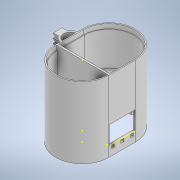
# Autodesk Inventor part: base-final
Saved by Autodesk Inventor 2021 (Build 250183000, 183)
## iProperties
Created: 2021-01-26
Part Number: base-final
Material: Generic
Document SubType Name: Modeling
Designer: Kayla
Density: 1 g/cm^3
Appearance: Default
Author: Kayla
Autodesk Inventor part; units mm, degrees
ref_plane "YZ Plane" through (0, 0, 0) normal (1, 0, 0) x (0, 1, 0)
ref_plane "XZ Plane" through (0, 0, 0) normal (0, 1, 0) x (-1, 0, 0)
ref_plane "XY Plane" through (0, 0, 0) normal (0, 0, 1) x (1, 0, 0)
sketch "Sketch1" plane through (0, 0, 0) normal (0, 1, 0) x (-1, 0, 0)
  line L0 (0, 0) -> (0, -60) construction
  line L1 (-60, 0) -> (-60, -60)
  line L2 (60, -60) -> (60, 0)
  arc A0 (60, 0) -> (-60, 0) centre (0, 0) ccw
  arc A1 (-60, -60) -> (60, -60) centre (0, -60) ccw
  point P0 (0, -30)
  dimension "d0" = 60
  dimension "d1" = 60
  constraints: 8 end point, 4 point on circle, 4 tangent, 2 centre point, 1 midpoint, 1 parallel, 1 vertical
  measures "d0" distance of L2.start L2.end
  measures "d1" radius of A1
extrude "Extrusion1" add sketch "Sketch1" along normal blind 160
sketch "Sketch2" plane through (0, 160, 0) normal (0, 1, 0) x (1, 0, 0)
  line L0 (0, 0) -> (0, 60) construction
  line L1 (56, 0) -> (56, 60)
  line L2 (-56, 60) -> (-56, 0)
  arc A0 (-56, 0) -> (56, 0) centre (0, 0) ccw
  arc A1 (56, 60) -> (-56, 60) centre (0, 60) ccw
  line L3 (-60, 60) -> (-60, 0) projected
  point P0 (0, 30)
  dimension "d5" = 4
  constraints: 8 end point, 4 point on circle, 4 tangent, 2 centre point, 1 midpoint, 1 parallel, 1 vertical
  measures "d5" distance between parallel lines of L3 L2
extrude "Extrusion2" cut sketch "Sketch2" against normal blind 86
sketch "Sketch3" plane through (0, 0, 0) normal (0, -1, 0) x (1, 0, 0)
  line L0 (0, 0) -> (0, -60) construction
  line L1 (-56, 0) -> (-56, -60)
  line L2 (56, -60) -> (56, 0)
  arc A0 (56, 0) -> (-56, 0) centre (0, 0) ccw
  arc A1 (-56, -60) -> (56, -60) centre (0, -60) ccw
  line L3 (60, 0) -> (60, -60) projected
  point P0 (0, -30)
  dimension "d8" = 4
  dimension "d9" = 60
  constraints: 8 end point, 4 point on circle, 4 tangent, 2 centre point, 1 midpoint, 1 parallel, 1 vertical
  measures "d8" distance between parallel lines of L3 L2
  measures "d9" distance of L2.start L2.end
extrude "Extrusion3" cut sketch "Sketch3" against normal blind 70
sketch "Sketch5" plane through (0, 160, 0) normal (0, 1, 0) x (1, 0, 0)
  arc A0 (-55.9943, 0) -> (55.9943, 0) centre (0, 0.0936) ccw
  line L0 (-55.9943, 0) -> (55.9943, 0)
  point P0 (0, 0)
  dimension "d14" = 111.9886
  constraints: 2 end point, 2 point on circle, 1 centre point, 1 horizontal
  measures "d14" distance of L0.end L0.start
extrude "Extrusion4" cut sketch "Sketch5" against normal blind 100
sketch "Sketch6" plane through (0, 74, 0) normal (0, 1, 0) x (1, 0, 0)
  line L0 (-56.7838, 0) -> (56.3732, 0)
  line L1 (56.3732, 0) -> (56.3732, 4)
  line L2 (56.3732, 4) -> (-56.7838, 4)
  line L3 (-56.7838, 4) -> (-56.7838, 0)
  point P0 (0, 0)
  dimension "d17" = 113.157
  dimension "d18" = 4
  constraints: 8 end point, 2 parallel, 1 horizontal, 1 perpendicular
  measures "d17" distance of L0.start L0.end
  measures "d18" distance of L2.end L0.start
extrude "Extrusion5" add sketch "Sketch6" along normal blind 86 and the other way blind 74
sketch "Sketch7" plane through (0, 0, 0) normal (0, -1, 0) x (1, 0, 0)
  arc A0 (57.3927, 0) -> (-56.9073, 0) centre (0.2427, -0.2605) ccw
  line L0 (57.3927, 0) -> (-56.9073, 0)
  point P0 (0, 0)
  dimension "d23" = 114.3
  constraints: 2 end point, 2 point on circle, 1 centre point, 1 horizontal
  measures "d23" distance of L0.end L0.start
extrude "Extrusion6" add sketch "Sketch7" against normal blind 4
sketch "Sketch8" plane through (0, 160, 0) normal (0, 1, 0) x (1, 0, 0)
  arc A0 (-56, 50) -> (-56, 10) centre (-56, 30) ccw
  line L0 (-56, 10) -> (-56, 50)
  arc A1 (60, 60) -> (-60, 60) centre (0, 60) ccw projected
  arc A2 (-60, 45.4919) -> (-60, 14.5081) centre (-56, 30) ccw
  line L1 (-60, 45.4919) -> (-60, 14.5081)
  line L2 (-56, 4) -> (-56, 60) projected
  point P0 (0, 0)
  dimension "d27" = 30
  dimension "d28" = 40
  dimension "d29" = 20
  dimension "d37" = 4
  dimension "d38" = 0
  constraints: 4 end point, 4 point on circle, 2 centre point, 1 vertical, 1 other
  measures "d27" vertical distance of A1.centre A0.centre
  measures "d28" distance of L0.start L0.end
  measures "d29" radius of A0
  measures "d37" distance between parallel lines of L0 L1
  measures "d38" distance between parallel lines of L2 L0
extrude "Extrusion7" add sketch "Sketch8" against normal blind 160
sketch "Sketch11" plane through (0, 0, 0) normal (0, -1, 0) x (1, 0, 0)
  line L0 (-60, -45.4919) -> (-56, -45.4919)
  line L1 (-56, -45.4919) -> (-56, -14.5081)
  line L2 (-56, -14.5081) -> (-60, -14.5081)
  line L3 (-60, -14.5081) -> (-60, -45.4919)
  line L4 (-60, -45.4919) -> (-60, -14.5081) projected
  point P0 (0, 0)
  dimension "d43" = 4
  dimension "d45" = 0
  dimension "d46" = 0
  dimension "d48" = 0
  constraints: 8 end point, 2 parallel, 1 horizontal, 1 perpendicular
  measures "d43" distance of L0.start L0.end
  measures "d45" distance between parallel lines of L4 L3
  measures "d46" distance from line of L0 L4.start
  measures "d48" distance from line of L2 L4.end
extrude "Extrusion8" cut sketch "Sketch11" against normal blind 50
sketch "Sketch12" plane through (0, 0, 0) normal (0, -1, 0) x (1, 0, 0)
  line L0 (-5, -4) -> (5, -4)
  line L1 (5, -4) -> (5, -14)
  line L2 (5, -14) -> (-5, -14)
  line L3 (-5, -14) -> (-5, -4)
  line L4 (-56, -4) -> (56, -4) projected
  line L5 (-5, -106) -> (5, -106)
  line L6 (5, -106) -> (5, -117)
  line L7 (5, -117) -> (-5, -117)
  line L8 (-5, -117) -> (-5, -106)
  arc A0 (-60, -60) -> (60, -60) centre (0, -60) ccw projected
  arc A1 (-56, -60) -> (56, -60) centre (0, -60) ccw
  point P0 (0, 0)
  point P1 (-5, -115.7763)
  point P2 (5, -115.7763)
  dimension "d51" = 10
  dimension "d52" = 10
  dimension "d53" = 0
  dimension "d54" = 5
  dimension "d55" = 11
  dimension "d56" = 10
  dimension "d57" = 5
  dimension "d58" = 3
  dimension "d63" = 56
  constraints: 16 end point, 4 parallel, 2 horizontal, 2 perpendicular, 2 point on circle, 1 centre point, 1 concentric
  measures "d51" distance of L2.end L0.start
  measures "d52" distance of L1.end L2.end
  measures "d53" distance between parallel lines of L4 L0
  measures "d54" distance from line of point (0, 0) L3
  measures "d55" distance of L7.end L5.start
  measures "d56" distance of L6.end L7.end
  measures "d57" distance from line of L8 point (0, 0)
  measures "d58" distance edge to line of A0 L7
  measures "d63" radius of A1
extrude "Extrusion11" add sketch "Sketch12" against normal blind 12.5 contours L0 L1 L2 L3 | L5 L6 A1 L8
extrude "Extrusion12" cut sketch "Sketch12" against normal blind 2 contours L0 L1 L2 L3 | L5 L6 A1 L8
sketch "Sketch16" plane through (0, 0, 0) normal (0, 0, 1) x (1, 0, 0)
  point P0 (0, 0)
sketch "Sketch17" plane through (0, 160, 0) normal (0, 1, 0) x (1, 0, 0)
  point P0 (0, 0)
sketch "Sketch18" plane through (60, 0, 0) normal (1, 0, 0) x (0, 0, -1)
  line L0 (1.5, 63.3446) -> (58.5, 63.3446)
  line L1 (58.5, 63.3446) -> (58.5, 22.3446)
  line L2 (58.5, 22.3446) -> (1.5, 22.3446)
  line L3 (1.5, 22.3446) -> (1.5, 63.3446)
  line L4 (0, 0) -> (0, 160) projected
  line L5 (60, 0) -> (60, 160) projected
  dimension "d68" = 57
  dimension "d69" = 41
  dimension "d72" = 1.5
  constraints: 8 end point, 2 parallel, 1 horizontal, 1 perpendicular
  measures "d68" distance of L0.start L0.end
  measures "d69" distance of L2.end L0.start
  measures "d72" distance between parallel lines of L4 L3
extrude "Extrusion13" cut sketch "Sketch18" against normal blind 10
sketch "Sketch20" plane through (0, 2, 0) normal (0, -1, 0) x (1, 0, 0)
  point P0 (0, 0)
  point P1 (-0.0272, -8.8829)
hole "Hole1" at (-0.0272, 2, -8.8829) direction (0, 1, 0) diameter 3 depth 15 tip angle 118
sketch "Sketch21" plane through (0, 2, 0) normal (0, -1, 0) x (1, 0, 0)
  point P0 (0, 0)
  point P1 (0.0411, -111.0492)
hole "Hole2" at (0.0411, 2, -111.0492) direction (0, 1, 0) diameter 3 depth 15 tip angle 118
sketch "Sketch22" plane through (0, 0, 0) normal (0, -1, 0) x (1, 0, 0)
  line L0 (-56, -14.5079) -> (-60, -14.5079)
  line L1 (-60, -45.4919) -> (-56, -45.4919)
  line L2 (-56, -45.4919) -> (-56, -14.5079)
  line L3 (-56, -45.4919) -> (-60, -45.4919) projected
  line L4 (-56, -14.5081) -> (-56, -45.4919) projected
  arc A0 (-60, -14.5079) -> (-60, -45.4919) centre (-56.0023, -29.9999) ccw
  arc A1 (-60, -14.5081) -> (-60, -45.4919) centre (-56, -30) ccw projected
  point P0 (0, 0)
  dimension "d90" = 30.984
  dimension "d91" = 0
  dimension "d92" = 4
  dimension "d93" = 0
  dimension "d94" = 0.0001
  constraints: 6 end point, 2 point on circle, 1 centre point, 1 horizontal, 1 parallel
  measures "d90" distance of L1.end L0.start
  measures "d91" distance between parallel lines of L3 L1
  measures "d92" distance of L1.start L1.end
  measures "d93" distance between parallel lines of L4 L2
  measures "d94" vertical distance of A1.centre A0.centre
extrude "Extrusion14" add sketch "Sketch22" against normal blind 4
sketch "Sketch23" plane through (0, 0, 0) normal (0, 0, 1) x (1, 0, 0)
  line L0 (-73.2, 160) -> (-85.2, 160)
  line L1 (-85.2, 160) -> (-85.2, 154)
  line L2 (-85.2, 154) -> (-73.2, 154)
  line L3 (-73.2, 154) -> (-73.2, 160)
  line L4 (-60, 160) -> (-76, 160) projected
  line L5 (-85.2, 150) -> (-73.2, 150)
  line L6 (-73.2, 150) -> (-73.2, 144)
  line L7 (-73.2, 144) -> (-85.2, 144)
  line L8 (-85.2, 144) -> (-85.2, 150)
  line L9 (-85.2, 140) -> (-73.2, 140)
  line L10 (-73.2, 140) -> (-73.2, 134)
  line L11 (-73.2, 134) -> (-85.2, 134)
  line L12 (-85.2, 134) -> (-85.2, 140)
  line L13 (-85.2, 130) -> (-73.2, 130)
  line L14 (-73.2, 130) -> (-73.2, 124)
  line L15 (-73.2, 124) -> (-85.2, 124)
  line L16 (-85.2, 124) -> (-85.2, 130)
  line L17 (-85.2, 120) -> (-73.2, 120)
  line L18 (-73.2, 120) -> (-73.2, 114)
  line L19 (-73.2, 114) -> (-85.2, 114)
  line L20 (-85.2, 114) -> (-85.2, 120)
  line L21 (-85.2, 110) -> (-73.2, 110)
  line L22 (-73.2, 110) -> (-73.2, 104)
  line L23 (-73.2, 104) -> (-85.2, 104)
  line L24 (-85.2, 104) -> (-85.2, 110)
  line L25 (-85.2, 100) -> (-73.2, 100)
  line L26 (-73.2, 100) -> (-73.2, 94)
  line L27 (-73.2, 94) -> (-85.2, 94)
  line L28 (-85.2, 94) -> (-85.2, 100)
  line L29 (-85.2, 90) -> (-73.2, 90)
  line L30 (-73.2, 90) -> (-73.2, 84)
  line L31 (-73.2, 84) -> (-85.2, 84)
  line L32 (-85.2, 84) -> (-85.2, 90)
  line L33 (-85.2, 80) -> (-73.2, 80)
  line L34 (-73.2, 80) -> (-73.2, 74)
  line L35 (-73.2, 74) -> (-85.2, 74)
  line L36 (-85.2, 74) -> (-85.2, 80)
  line L37 (-85.2, 70) -> (-73.2, 70)
  line L38 (-73.2, 70) -> (-73.2, 64)
  line L39 (-73.2, 64) -> (-85.2, 64)
  line L40 (-85.2, 64) -> (-85.2, 70)
  line L41 (-60, 0) -> (-60, 160) projected
  point P0 (0, 0)
  dimension "d97" = 0
  dimension "d98" = 6
  dimension "d99" = 12
  dimension "d100" = 12
  dimension "d101" = 6
  dimension "d102" = 4
  dimension "d103" = 12
  dimension "d104" = 6
  dimension "d105" = 4
  dimension "d106" = 12
  dimension "d107" = 6
  dimension "d108" = 4
  dimension "d109" = 12
  dimension "d110" = 6
  dimension "d111" = 4
  dimension "d112" = 12
  dimension "d113" = 6
  dimension "d114" = 4
  dimension "d115" = 12
  dimension "d116" = 6
  dimension "d117" = 4
  dimension "d118" = 12
  dimension "d119" = 6
  dimension "d120" = 4
  dimension "d121" = 6
  dimension "d122" = 4
  dimension "d123" = 12
  dimension "d124" = 12
  dimension "d125" = 6
  dimension "d126" = 4
  dimension "d136" = 13.2
  dimension "d137" = 13.2
  constraints: 80 end point, 20 parallel, 10 horizontal, 10 perpendicular
  measures "d97" distance between parallel lines of L4 L0
  measures "d98" distance of L0.end L1.end
  measures "d99" distance of L0.start L0.end
  measures "d100" distance of L5.start L5.end
  measures "d101" distance of L7.end L5.start
  measures "d102" distance between parallel lines of L5 L2
  measures "d103" distance of L9.start L9.end
  measures "d104" distance of L11.end L9.start
  measures "d105" distance between parallel lines of L7 L9
  measures "d106" distance of L13.start L13.end
  measures "d107" distance of L15.end L13.start
  measures "d108" distance between parallel lines of L11 L13
  measures "d109" distance of L17.start L17.end
  measures "d110" distance of L19.end L17.start
  measures "d111" distance between parallel lines of L15 L17
  measures "d112" distance of L21.start L21.end
  measures "d113" distance of L23.end L21.start
  measures "d114" distance between parallel lines of L19 L21
  measures "d115" distance of L25.start L25.end
  measures "d116" distance of L27.end L25.start
  measures "d117" distance between parallel lines of L23 L25
  measures "d118" distance of L29.start L29.end
  measures "d119" distance of L31.end L29.start
  measures "d120" distance between parallel lines of L27 L29
  measures "d121" distance of L35.end L33.start
  measures "d122" distance between parallel lines of L31 L33
  measures "d123" distance of L33.start L33.end
  measures "d124" distance of L37.start L37.end
  measures "d125" distance of L39.end L37.start
  measures "d126" distance between parallel lines of L35 L37
  measures "d136" distance between parallel lines of L41 L3
  measures "d137" distance between parallel lines of L41 L6
extrude "Extrusion15" add sketch "Sketch23" against normal blind 40
extrude "Extrusion16" cut sketch "Sketch23" against normal blind 20
chamfer "Chamfer1" distance 5 angle 45 10 edges at (-85.2, 154, -30) (-85.2, 144, -30) (-85.2, 134, -30) (-85.2, 124, -30) (-85.2, 114, -30) (-85.2, 104, -30) (-85.2, 94, -30) (-85.2, 84, -30) (-85.2, 74, -30) (-85.2, 64, -30)
sketch "Sketch26" plane through (60, 22.3446, -1.5) normal (0, 0, -1) x (-1, 0, 0)
  line L0 (7.4, 41.6149) -> (3.4, 41.6149)
  line L1 (3.4, 41.6149) -> (3.4, 0.0149)
  line L2 (3.4, 0.0149) -> (7.4, 0.0149)
  line L3 (7.4, 0.0149) -> (7.4, 41.6149)
  line L4 (0, 0) -> (0, 41) projected
  line L5 (120, -22.3446) -> (0, -22.3446) projected
  point P0 (60, -22.3446)
  dimension "d140" = 3.4
  dimension "d141" = 4
  dimension "d190" = 22.3594
  dimension "d191" = 41.6
  constraints: 8 end point, 2 parallel, 1 horizontal, 1 perpendicular
  measures "d140" distance between parallel lines of L4 L1
  measures "d141" distance between parallel lines of L1 L3
  measures "d190" distance between parallel lines of L5 L2
  measures "d191" distance between parallel lines of L0 L2
extrude "Extrusion17" cut sketch "Sketch26" against normal blind 9
sketch "Sketch27" plane through (52.6, 22.3594, -1.5) normal (0, 1, 0) x (1, 0, 0)
  line L0 (0, 0) -> (4, 0) projected
  line L1 (3.4, -1.5) -> (0, -1.5) projected
  line L2 (7.4, 57) -> (7.4, 0) projected
  point P0 (-52.6, -1.5)
sketch "Sketch28" plane through (-56, 160, 0) normal (0, 0, 1) x (1, 0, 0)
  line L0 (111.9993, -95.1493) -> (108.6, -95.1493)
  line L1 (108.6, -95.1493) -> (108.6, -94.1493)
  line L2 (108.6, -94.1493) -> (111.9993, -94.1493)
  line L3 (111.9993, -94.1493) -> (111.9993, -95.1493)
  line L4 (108.6, -94.1493) -> (107.6, -94.1493)
  line L5 (107.6, -94.1493) -> (107.6, -137.6406)
  line L6 (107.6, -137.6406) -> (108.6, -137.6406)
  line L7 (108.6, -137.6406) -> (108.6, -94.1493)
  line L8 (111.9993, -137.6406) -> (107.6, -137.6406)
  line L9 (107.6, -137.6406) -> (107.6, -138.6406)
  line L10 (107.6, -138.6406) -> (111.9993, -138.6406)
  line L11 (111.9993, -138.6406) -> (111.9993, -137.6406)
  line L12 (108.6, -137.6406) -> (108.6, -96.0406) projected
  line L13 (112, -137.6406) -> (108.6, -137.6406) projected
  point P0 (56, -160)
  dimension "d149" = 1
  dimension "d150" = 0
  dimension "d151" = 1
  dimension "d152" = 0
  dimension "d189" = 1
  constraints: 24 end point, 6 parallel, 3 horizontal, 3 perpendicular, 3 point on line
  measures "d149" distance between parallel lines of L5 L7
  measures "d150" distance between parallel lines of L12 L7
  measures "d151" distance between parallel lines of L10 L8
  measures "d152" distance between parallel lines of L13 L8
  measures "d189" distance between parallel lines of L2 L0
extrude "Extrusion18" add sketch "Sketch28" along normal blind 20
sketch "Sketch29" plane through (60, 0, 0) normal (1, 0, 0) x (0, 0, -1)
  line L0 (26.8, 20.5733) -> (33.2, 20.5733)
  line L1 (33.2, 20.5733) -> (33.2, 14.1733)
  line L2 (33.2, 14.1733) -> (26.8, 14.1733)
  line L3 (26.8, 14.1733) -> (26.8, 20.5733)
  line L4 (48.2, 20.5733) -> (54.6, 20.5733)
  line L5 (54.6, 20.5733) -> (54.6, 14.1733)
  line L6 (54.6, 14.1733) -> (48.2, 14.1733)
  line L7 (48.2, 14.1733) -> (48.2, 20.5733)
  line L8 (5.4, 20.5733) -> (11.8, 20.5733)
  line L9 (11.8, 20.5733) -> (11.8, 14.1733)
  line L10 (11.8, 14.1733) -> (5.4, 14.1733)
  line L11 (5.4, 14.1733) -> (5.4, 20.5733)
  line L12 (60, 0) -> (60, 160) projected
  line L13 (0, 0) -> (0, 160) projected
  dimension "d155" = 6.4
  dimension "d156" = 6.4
  dimension "d157" = 6.4
  dimension "d158" = 6.4
  dimension "d159" = 6.4
  dimension "d160" = 6.4
  dimension "d161" = 60
  dimension "d162" = 26.8
  dimension "d163" = 15
  dimension "d164" = 15
  dimension "d165" = 0
  constraints: 24 end point, 6 parallel, 3 horizontal, 3 perpendicular, 1 point on line
  measures "d155" distance of L8.start L8.end
  measures "d156" distance of L10.end L8.start
  measures "d157" distance of L0.start L0.end
  measures "d158" distance of L2.end L0.start
  measures "d159" distance of L4.start L4.end
  measures "d160" distance of L6.end L4.start
  measures "d161" distance between parallel lines of L12 L13
  measures "d162" distance between parallel lines of L13 L3
  measures "d163" distance between parallel lines of L3 L9
  measures "d164" distance between parallel lines of L1 L7
  measures "d165" distance between parallel lines of L0 L8
extrude "Extrusion19" cut sketch "Sketch29" against normal blind 5
sketch "Sketch30" plane through (60, 22.3446, -58.5) normal (0, 0, 1) x (1, 0, 0)
  line L0 (-4.0085, 41.0021) -> (-3.4, 41.0021)
  line L1 (-3.4, 41.0021) -> (-3.4, 0.0001)
  line L2 (-3.4, 0.0001) -> (-4.0085, 0.0001)
  line L3 (-4.0085, 0.0001) -> (-4.0085, 41.0021)
  line L4 (0, 41) -> (0, 0) projected
  point P0 (-60, -22.3446)
  dimension "d170" = 3.4
  constraints: 8 end point, 2 parallel, 1 horizontal, 1 perpendicular
  measures "d170" distance between parallel lines of L1 L4
extrude "Extrusion20" cut sketch "Sketch30" against normal blind 9
sketch "Sketch31" plane through (0, 160, 0) normal (0, 1, 0) x (1, 0, 0)
  line L0 (-56, 4) -> (56, 4)
  line L1 (-56, 4) -> (-56, 60) projected
  line L2 (56, 60) -> (56, 4) projected
  line L3 (56, 4) -> (-56, 4) projected
  arc A0 (56, 60) -> (-56, 60) centre (0, 60) ccw
  arc A1 (-56, 0) -> (56, 0) centre (0, 0) ccw
  arc A2 (57.6, 60) -> (-57.6, 60) centre (0, 60) ccw
  arc A3 (60, 60) -> (-60, 60) centre (0, 60) ccw projected
  arc A4 (-57.6, 0) -> (57.6, 0) centre (0, 0) ccw
  line L4 (-57.6, 0) -> (57.6, 0)
  line L5 (57.6, 0) -> (57.6, 4)
  line L6 (57.6, 4) -> (-57.6, 4)
  line L7 (-57.6, 4) -> (-57.6, 0)
  line L8 (-57.6, 4) -> (-57.6, 60)
  line L9 (-56, 4) -> (-56, 60)
  line L10 (57.6, 4) -> (57.6, 60)
  line L11 (56, 4) -> (56, 60)
  point P0 (0, 0)
  point P1 (57.6, 0)
  point P2 (56, 0)
  point P3 (56, 4)
  dimension "d176" = 0
  dimension "d177" = 112
  dimension "d181" = 1.6
  dimension "d182" = 1.6
  constraints: 18 end point, 8 point on circle, 6 equal length, 4 centre point, 2 horizontal, 2 tangent, 1 perpendicular, 1 point on line
  measures "d176" distance between parallel lines of L3 L0
  measures "d177" distance of A1.start A1.end
  measures "d181" radial gap between concentric circles of A2 A0
  measures "d182" radial gap between concentric circles of A4 A1
extrude "Extrusion21" cut sketch "Sketch31" against normal blind 10 contours L4 A1 A4
extrude "Extrusion22" cut sketch "Sketch31" against normal blind 10 contours L6 L8 A2 L10 L2 A0 L1
sketch "Sketch33" plane through (60, 63.3446, -58.5) normal (0, -1, 0) x (1, 0, 0)
  line L0 (-10, 54.5) -> (-3.4, 54.5)
  line L1 (-3.4, 54.5) -> (-3.4, 57)
  line L2 (-3.4, 57) -> (-10, 57)
  line L3 (-10, 57) -> (-10, 54.5)
  line L4 (-4, 0) -> (-4, 54.5) projected
  line L5 (-3.4, 57) -> (-7.4, 57) projected
  line L6 (-4, 54.5) -> (-10, 54.5) projected
  line L7 (-10, 57) -> (-10, 54.5) projected
  line L8 (-3.4, 54.5) -> (-4, 54.5)
  line L9 (-4, 54.5) -> (-4, 0)
  line L10 (-4, 0) -> (-3.4, 0)
  line L11 (-3.4, 0) -> (-3.4, 54.5)
  line L12 (0, 0) -> (-3.4, 0) projected
  point P0 (-60, 58.5)
  dimension "d193" = 0
  dimension "d194" = 0
  dimension "d195" = 0
  dimension "d196" = 0
  dimension "d197" = 0
  constraints: 16 end point, 4 parallel, 2 horizontal, 2 perpendicular, 1 point on line
  measures "d193" distance between parallel lines of L5 L2
  measures "d194" distance between parallel lines of L6 L0
  measures "d195" distance between parallel lines of L7 L3
  measures "d196" distance from line of L5.start L1
  measures "d197" distance between parallel lines of L12 L10
extrude "Extrusion23" cut sketch "Sketch33" against normal blind 0.6
body "Solid1"
